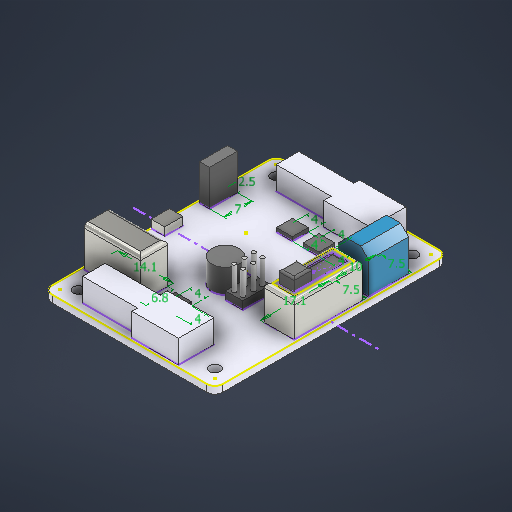
# Autodesk Inventor part: SERIAL_BUS_SERVO_CONTROLLER
Saved by Autodesk Inventor 2027.1 (Build 311270010, 270A)
## iProperties
Created: 2026-08-16
Part Number: SERIAL_BUS_SERVO_CONTROLLER
Material: Genérico
Document SubType Name: Modeling
Designer: Evellyn
Density: 1 g/cm^3
Appearance: Padrão
Author: Evellyn
Autodesk Inventor part; units mm, degrees
ref_plane "YZ Plane" through (0, 0, 0) normal (1, 0, 0) x (0, 1, 0)
ref_plane "XZ Plane" through (0, 0, 0) normal (0, 1, 0) x (-1, 0, 0)
ref_plane "XY Plane" through (0, 0, 0) normal (0, 0, 1) x (1, 0, 0)
sketch "Esboço1" plane through (0, 0, 0) normal (0, 1, 0) x (-1, 0, 0)
  line L0 (-19.4, -29.1) -> (19.4, -29.1)
  line L1 (21.4, -27.1) -> (21.4, 27.1)
  line L2 (19.4, 29.1) -> (-19.4, 29.1)
  line L3 (-21.4, 27.1) -> (-21.4, -27.1)
  line L4 (-21.4, -29.1) -> (21.4, 29.1) construction
  line L5 (21.4, -29.1) -> (-21.4, 29.1) construction
  circle A0 centre (17.05, 24.75) radius 1.35
  circle A1 centre (-17.05, 24.75) radius 1.35
  circle A2 centre (17.05, -24.75) radius 1.35
  circle A3 centre (-17.05, -24.75) radius 1.35
  arc A4 (21.4, 27.1) -> (19.4, 29.1) centre (19.4, 27.1) ccw
  arc A5 (-19.4, 29.1) -> (-21.4, 27.1) centre (-19.4, 27.1) ccw
  arc A6 (19.4, -29.1) -> (21.4, -27.1) centre (19.4, -27.1) ccw
  arc A7 (-21.4, -27.1) -> (-19.4, -29.1) centre (-19.4, -27.1) ccw
  point P0 (0, 0)
  dimension "d0" = 42.8
  dimension "d1" = 58.2
  dimension "d2" = 2.7
  dimension "d3" = 3
  dimension "d4" = 3
  dimension "d5" = 2.7
  dimension "d6" = 3
  dimension "d7" = 3
  dimension "d8" = 2
  dimension "d57" = 34.1
  dimension "d58" = 34.1
  dimension "d59" = 49.5
  dimension "d60" = 49.5
  constraints: 12 end point, 8 centre point, 8 point on circle, 8 point on line, 8 tangent, 3 equal radius, 2 midpoint, 2 parallel, 1 horizontal, 1 perpendicular
  measures "d0" distance of L5.end L4.end
  measures "d1" distance of L4.end L5.start
  measures "d2" diameter of A0
  measures "d3" distance edge to line of A0 L1
  measures "d4" distance edge to line of A0 L2
  measures "d5" diameter of A1
  measures "d6" distance edge to line of A1 L3
  measures "d7" distance edge to line of A1 L2
  measures "d8" radius of A4
  measures "d57" distance of A3.centre A2.centre
  measures "d58" distance of A1.centre A0.centre
  measures "d59" distance of A0.centre A2.centre
  measures "d60" distance of A1.centre A3.centre
extrude "Extrusão1" add sketch "Esboço1" along normal blind 1.8
sketch "Esboço2" plane through (0, 1.8, 0) normal (0, 1, 0) x (1, 0, 0)
  line L0 (-21.4, 27.1) -> (-21.4, -27.1) projected
  arc A0 (-21.4, -27.1) -> (-19.4, -29.1) centre (-19.4, -27.1) ccw projected
  arc A1 (-19.4, 29.1) -> (-21.4, 27.1) centre (-19.4, 27.1) ccw projected
  line L1 (19.4, 29.1) -> (-19.4, 29.1) projected
  line L2 (-19.4, -29.1) -> (19.4, -29.1) projected
  arc A2 (19.4, -29.1) -> (21.4, -27.1) centre (19.4, -27.1) ccw projected
  line L3 (21.4, -27.1) -> (21.4, 27.1) projected
  arc A3 (21.4, 27.1) -> (19.4, 29.1) centre (19.4, 27.1) ccw projected
  line L4 (20.7322, -8.55) -> (13.2322, -8.55)
  line L5 (13.2322, -8.55) -> (13.2322, 8.55)
  line L6 (13.2322, 8.55) -> (20.7322, 8.55)
  line L7 (20.7322, 8.55) -> (20.7322, -8.55)
  line L8 (20.7322, -8.55) -> (13.2322, 8.55) construction
  line L9 (13.2322, -8.55) -> (20.7322, 8.55) construction
  line L10 (20.7322, 10.1228) -> (13.2322, 10.1228)
  line L11 (13.2322, 10.1228) -> (13.2322, 20.1228)
  line L12 (13.2322, 20.1228) -> (20.7322, 20.1228)
  line L13 (20.7322, 20.1228) -> (20.7322, 10.1228)
  line L14 (-20.8142, -19.6445) -> (-6.7142, -19.6445)
  line L15 (-6.7142, -19.6445) -> (-6.7142, -12.8445)
  line L16 (-6.7142, -12.8445) -> (-20.8142, -12.8445)
  line L17 (-20.8142, -12.8445) -> (-20.8142, -19.6445)
  line L18 (-28.189, 0) -> (33.4078, 0)
  line L19 (-21.4, -2.2988) -> (-18.0103, -2.2988)
  line L20 (-18.0103, -2.2988) -> (-18.0103, 2.2923)
  line L21 (-18.0103, 2.2923) -> (-21.4, 2.2923)
  line L22 (-21.4, 2.2923) -> (-21.4, -2.2988)
  line L23 (-13.7642, -27.1) -> (0, -27.1)
  line L24 (0, -21.4359) -> (-13.7642, -21.4359)
  line L25 (-13.7642, -21.4359) -> (-13.7642, -27.1)
  line L26 (0, -28.5142) -> (11.7075, -28.5142)
  line L27 (11.7075, -28.5142) -> (11.7075, -19.6445)
  line L28 (11.7075, -19.6445) -> (0, -19.6445)
  line L29 (0, -19.6445) -> (0, -21.4359)
  line L30 (0, -27.1) -> (0, -28.5142)
  line L31 (-13.7642, 27.1) -> (0, 27.1)
  line L32 (0, 21.4359) -> (-13.7642, 21.4359)
  line L33 (-13.7642, 21.4359) -> (-13.7642, 27.1)
  line L34 (0, 28.5142) -> (11.7075, 28.5142)
  line L35 (11.7075, 28.5142) -> (11.7075, 19.6445)
  line L36 (11.7075, 19.6445) -> (0, 19.6445)
  line L37 (0, 19.6445) -> (0, 21.4359)
  line L38 (0, 27.1) -> (0, 28.5142)
  line L39 (3.5052, -8.55) -> (7.8476, -8.55)
  line L40 (7.8476, -8.55) -> (7.8476, -1.4997)
  line L41 (7.8476, -1.4997) -> (3.5052, -1.4997)
  line L42 (3.5052, -1.4997) -> (3.5052, -8.55)
  circle A4 centre (0, -5.0249) radius 3.428
  line L43 (-3.428, -18.1455) -> (0.572, -18.1455)
  line L44 (0.572, -18.1455) -> (0.572, -14.1455)
  line L45 (0.572, -14.1455) -> (-3.428, -14.1455)
  line L46 (-3.428, -14.1455) -> (-3.428, -18.1455)
  line L47 (-4.8578, 12.5931) -> (-0.8578, 12.5931)
  line L48 (-0.8578, 12.5931) -> (-0.8578, 16.5931)
  line L49 (-0.8578, 16.5931) -> (-4.8578, 16.5931)
  line L50 (-4.8578, 16.5931) -> (-4.8578, 12.5931)
  line L51 (1.8165, 12.5931) -> (5.8165, 12.5931)
  line L52 (5.8165, 12.5931) -> (5.8165, 16.5931)
  line L53 (5.8165, 16.5931) -> (1.8165, 16.5931)
  line L54 (1.8165, 16.5931) -> (1.8165, 12.5931)
  line L55 (-20.8142, 9.2758) -> (-18.3142, 9.2758)
  line L56 (-18.3142, 9.2758) -> (-18.3142, 16.2758)
  line L57 (-18.3142, 16.2758) -> (-20.8142, 16.2758)
  line L58 (-20.8142, 16.2758) -> (-20.8142, 9.2758)
  point P0 (0, 0)
  point P1 (16.9822, 0)
  dimension "d11" = 7.5
  dimension "d12" = 17.1
  dimension "d13" = 7.5
  dimension "d14" = 10
  dimension "d15" = 14.1
  dimension "d16" = 6.8
  dimension "d17" = 4
  dimension "d18" = 4
  dimension "d19" = 4
  dimension "d20" = 4
  dimension "d21" = 4
  dimension "d22" = 4
  dimension "d23" = 2.5
  dimension "d24" = 7
  constraints: 110 end point, 22 parallel, 12 horizontal, 10 perpendicular, 8 symmetric about line, 2 midpoint, 1 centre point, 1 point on line
  measures "d11" distance of L5.end L6.end
  measures "d12" distance of L4.end L5.end
  measures "d13" distance of L11.end L12.end
  measures "d14" distance of L10.end L11.end
  measures "d15" distance of L16.end L15.end
  measures "d16" distance of L15.end L14.end
  measures "d17" distance of L45.end L44.end
  measures "d18" distance of L44.end L43.end
  measures "d19" distance of L49.end L48.end
  measures "d20" distance of L48.end L47.end
  measures "d21" distance of L53.end L52.end
  measures "d22" distance of L52.end L51.end
  measures "d23" distance of L57.end L56.end
  measures "d24" distance of L56.end L55.end
extrude "Extrusão2" add sketch "Esboço2" along normal blind 8.5 contours L18 L7 L4 L5 | L5 L6 L7 L18
extrude "Extrusão3" add sketch "Esboço2" along normal blind 10 contours L10 L11 L12 L13 | L17 L16 L15 L14
extrude "Extrusão4" add sketch "Esboço2" along normal blind 5.8 contours L25 L24 L29 L28 L27 L26 L30 L23 | L31 L38 L34 L35 L36 L37 L32 L33
extrude "Extrusão5" add sketch "Esboço2" along normal blind 1 contours L46 L45 L44 L43 | L50 L49 L48 L47 | L54 L53 L52 L51
extrude "Extrusão6" add sketch "Esboço2" along normal blind 2 contours L21 L20 L18 L0 | L18 L20 L19 L0 | L42 L41 L40 L39
extrude "Extrusão7" add sketch "Esboço2" along normal blind 9 contours L58 L57 L56 L55
extrude "Extrusão8" add sketch "Esboço2" along normal blind 6 contours A4
chamfer "Chanfro1" distance 2 angle 45 2 edges at (20.7322, 11.8, -15.1228) (13.2322, 11.8, -15.1228)
fillet "Arredondamento1" radius 1 4 edges at (20.7322, 10.3, 0) (13.2322, 10.3, 0) (16.9822, 10.3, 8.55) (16.9822, 10.3, -8.55)
fillet "Arredondamento2" radius 1 3 edges at (-13.7642, 11.8, 19.6445) (-13.7642, 11.8, 12.8445) (-6.7142, 11.8, 16.2445)
sketch "Esboço3" plane through (0, 3.8, 0) normal (0, 1, 0) x (1, 0, 0)
  line L0 (7.8476, -1.4997) -> (3.5052, -1.4997) projected
  line L1 (3.5052, -1.4997) -> (3.5052, -8.55) projected
  line L2 (7.8476, -8.55) -> (7.8476, -1.4997) projected
  line L3 (3.5052, -8.55) -> (7.8476, -8.55) projected
  line L4 (3.5052, -1.4997) -> (7.8476, -1.4997)
  line L5 (7.8476, -1.4997) -> (7.8476, -3.7821)
  line L6 (7.8476, -3.7821) -> (3.5052, -3.7821)
  line L7 (3.5052, -3.7821) -> (3.5052, -1.4997)
  line L8 (3.5052, -3.7821) -> (7.8476, -3.7821)
  line L9 (7.8476, -3.7821) -> (7.8476, -6.0999)
  line L10 (7.8476, -6.0999) -> (3.5052, -6.0999)
  line L11 (3.5052, -6.0999) -> (3.5052, -3.7821)
  line L12 (5.6764, -1.4997) -> (5.6764, -8.55)
  circle A0 centre (4.673, -2.6409) radius 0.5
  circle A1 centre (6.8599, -2.6409) radius 0.5
  circle A2 centre (4.673, -4.941) radius 0.5
  circle A3 centre (6.8599, -4.941) radius 0.5
  circle A4 centre (4.673, -7.5205) radius 0.5
  circle A5 centre (6.8599, -7.5205) radius 0.5
  point P0 (0, 0)
  dimension "d44" = 1
  dimension "d45" = 1
  dimension "d46" = 1
  dimension "d47" = 1
  dimension "d48" = 1
  dimension "d49" = 1
  constraints: 18 end point, 6 centre point, 4 parallel, 2 horizontal, 2 midpoint, 2 perpendicular, 2 point on line
  measures "d44" diameter of A0
  measures "d45" diameter of A1
  measures "d46" diameter of A2
  measures "d47" diameter of A3
  measures "d48" diameter of A4
  measures "d49" diameter of A5
extrude "Extrusão9" add sketch "Esboço3" along normal blind 6 contours A0 | A1 | A2 | A3 | A4 | A5
sketch "Esboço4" plane through (0, 10.3, 0) normal (0, 1, 0) x (1, 0, 0)
  line L0 (14.2322, 7.55) -> (19.7322, 7.55) projected
  line L1 (14.2322, -7.55) -> (14.2322, 7.55) projected
  line L2 (19.7322, 7.55) -> (19.7322, -7.55) projected
  line L3 (19.7322, -7.55) -> (14.2322, -7.55) projected
  line L4 (18.8699, -6.7178) -> (15.0945, -6.7178)
  line L5 (15.0945, -6.7178) -> (15.0945, 6.7178)
  line L6 (15.0945, 6.7178) -> (18.8699, 6.7178)
  line L7 (18.8699, 6.7178) -> (18.8699, -6.7178)
  line L8 (18.8699, -6.7178) -> (15.0945, 6.7178) construction
  line L9 (15.0945, -6.7178) -> (18.8699, 6.7178) construction
  line L10 (15.0945, -2.2873) -> (18.8699, -2.2873)
  line L11 (18.8699, -2.2873) -> (18.8699, -6.7178)
  line L12 (18.8699, -6.7178) -> (15.0945, -6.7178)
  line L13 (15.0945, -6.7178) -> (15.0945, -2.2873)
  point P0 (0, 0)
  point P1 (16.9822, 0)
  constraints: 20 end point, 4 parallel, 2 horizontal, 2 midpoint, 2 perpendicular, 1 point on line
extrude "Extrusão10" add sketch "Esboço4" along normal blind 3 contours L4 L5 L10 L7
extrude "Extrusão11" cut sketch "Esboço4" against normal blind 0.5 contours L10 L5 L6 L7
fillet "Arredondamento3" radius 0.5 4 edges at (16.9822, 13.3, 6.7178) (18.8699, 13.3, 4.5025) (16.9822, 13.3, 2.2873) (15.0945, 13.3, 4.5025)
